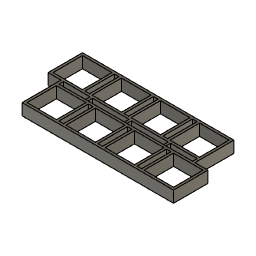
Macropad_V1_Plate (Autodesk Fusion 360 design; units mm, degrees)
Autodesk Fusion 360 part; units mm, degrees
sketch "Sketch1" plane through (0, 0, 0) normal (0, 0, 1) x (1, 0, 0)
  line L0 (0, 0) -> (80.3, 0)
  line L1 (80.3, 0) -> (80.3, 35.85)
  line L2 (80.3, 35.85) -> (0, 35.85)
  line L3 (0, 35.85) -> (0, 0)
  line L4 (1.2, 34.65) -> (15.6, 34.65)
  line L5 (15.6, 34.65) -> (15.6, 20.25)
  line L6 (15.6, 20.25) -> (1.2, 20.25)
  line L7 (1.2, 20.25) -> (1.2, 34.65)
  line L8 (20.25, 20.25) -> (20.25, 34.65)
  line L9 (20.25, 34.65) -> (34.65, 34.65)
  line L10 (34.65, 34.65) -> (34.65, 20.25)
  line L11 (34.65, 20.25) -> (20.25, 20.25)
  line L12 (39.3, 20.25) -> (39.3, 34.65)
  line L13 (39.3, 34.65) -> (53.7, 34.65)
  line L14 (53.7, 34.65) -> (53.7, 20.25)
  line L15 (53.7, 20.25) -> (39.3, 20.25)
  line L16 (58.35, 20.25) -> (58.35, 34.65)
  line L17 (58.35, 34.65) -> (72.75, 34.65)
  line L18 (72.75, 34.65) -> (72.75, 20.25)
  line L19 (72.75, 20.25) -> (58.35, 20.25)
  line L20 (7.55, 1.2) -> (7.55, 15.6)
  line L21 (7.55, 15.6) -> (21.95, 15.6)
  line L22 (21.95, 15.6) -> (21.95, 1.2)
  line L23 (21.95, 1.2) -> (7.55, 1.2)
  line L24 (26.6, 1.2) -> (26.6, 15.6)
  line L25 (26.6, 15.6) -> (41, 15.6)
  line L26 (41, 15.6) -> (41, 1.2)
  line L27 (41, 1.2) -> (26.6, 1.2)
  line L28 (45.65, 1.2) -> (45.65, 15.6)
  line L29 (45.65, 15.6) -> (60.05, 15.6)
  line L30 (60.05, 15.6) -> (60.05, 1.2)
  line L31 (60.05, 1.2) -> (45.65, 1.2)
  line L32 (64.7, 1.2) -> (64.7, 15.6)
  line L33 (64.7, 15.6) -> (79.1, 15.6)
  line L34 (79.1, 15.6) -> (79.1, 1.2)
  line L35 (79.1, 1.2) -> (64.7, 1.2)
  line L36 (19.05, 34.65) -> (16.8, 34.65)
  line L37 (16.8, 34.65) -> (16.8, 20.25)
  line L38 (16.8, 20.25) -> (19.05, 20.25)
  line L39 (19.05, 20.25) -> (19.05, 34.65)
  line L40 (35.85, 34.65) -> (35.85, 20.25)
  line L41 (35.85, 20.25) -> (38.1, 20.25)
  line L42 (38.1, 20.25) -> (38.1, 34.65)
  line L43 (38.1, 34.65) -> (35.85, 34.65)
  line L44 (54.9, 34.65) -> (54.9, 20.25)
  line L45 (54.9, 20.25) -> (57.15, 20.25)
  line L46 (57.15, 20.25) -> (57.15, 34.65)
  line L47 (57.15, 34.65) -> (54.9, 34.65)
  line L48 (25.4, 15.6) -> (23.15, 15.6)
  line L49 (23.15, 15.6) -> (23.15, 1.2)
  line L50 (23.15, 1.2) -> (25.4, 1.2)
  line L51 (25.4, 1.2) -> (25.4, 15.6)
  line L52 (42.2, 15.6) -> (42.2, 1.2)
  line L53 (42.2, 1.2) -> (44.45, 1.2)
  line L54 (44.45, 1.2) -> (44.45, 15.6)
  line L55 (44.45, 15.6) -> (42.2, 15.6)
  line L56 (61.25, 15.6) -> (61.25, 1.2)
  line L57 (61.25, 1.2) -> (63.5, 1.2)
  line L58 (63.5, 1.2) -> (63.5, 15.6)
  line L59 (63.5, 15.6) -> (61.25, 15.6)
  line L60 (72.75, 19.05) -> (7.55, 19.05)
  line L61 (7.55, 19.05) -> (7.55, 16.8)
  line L62 (7.55, 16.8) -> (72.75, 16.8)
  line L63 (72.75, 16.8) -> (72.75, 19.05)
  line L64 (80.3, 35.85) -> (73.95, 35.85)
  line L65 (73.95, 35.85) -> (73.95, 16.8)
  line L66 (73.95, 16.8) -> (80.3, 16.8)
  line L67 (80.3, 16.8) -> (80.3, 35.85)
  line L68 (0, 0) -> (6.35, 0)
  line L69 (6.35, 0) -> (6.35, 19.05)
  line L70 (6.35, 19.05) -> (0, 19.05)
  line L71 (0, 19.05) -> (0, 0)
  line L72 (21.7, 19.05) -> (20.5, 19.05)
  line L73 (20.5, 19.05) -> (20.5, 16.8018)
  line L74 (20.5, 16.8018) -> (21.7, 16.8018)
  line L75 (21.7, 16.8018) -> (21.7, 19.05)
  line L76 (40.75, 16.8018) -> (40.75, 19.05)
  line L77 (40.75, 19.05) -> (39.55, 19.05)
  line L78 (39.55, 19.05) -> (39.55, 16.8018)
  line L79 (39.55, 16.8018) -> (40.75, 16.8018)
  line L80 (59.8, 16.8018) -> (59.8, 19.05)
  line L81 (59.8, 19.05) -> (58.6, 19.05)
  line L82 (58.6, 19.05) -> (58.6, 16.8018)
  line L83 (58.6, 16.8018) -> (59.8, 16.8018)
  dimension "d6" = 14.4
  dimension "d7" = 14.4
  dimension "d12" = 19.05
  dimension "d13" = 0
  dimension "d14" = 14.4
  dimension "d15" = 14.4
  dimension "d16" = 19.05
  dimension "d17" = 6.35
  dimension "d20" = 19.05
  dimension "d21" = 0
  dimension "d22" = 1.2
  dimension "d23" = 1.2
  dimension "d24" = 1.2
  dimension "d25" = 1.2
  dimension "d37" = 1.2
  dimension "d39" = 1.2
  dimension "d42" = 19.05
  dimension "d43" = 0
  dimension "d45" = 1.2
  dimension "d46" = 1.2
  dimension "d49" = 19.05
  dimension "d50" = 0
  dimension "d54" = 1.2
  dimension "d55" = 1.2
  dimension "d57" = 1.2
  dimension "d59" = 1.2
  dimension "d60" = 1.2
  dimension "d61" = 0.25
  dimension "d64" = 19.05
  dimension "d65" = 0
  constraint horizontal L0
  constraint vertical L1
  constraint horizontal L2
  constraint vertical L3
  constraint coincident L0.start L3.end
  constraint horizontal L4
  constraint vertical L5
  constraint horizontal L6
  constraint vertical L7
  constraint horizontal L21
  constraint vertical L22
  constraint horizontal L23
  constraint vertical L20
  constraint horizontal L36
  constraint vertical L37
  constraint horizontal L38
  constraint vertical L39
  constraint collinear L4 L36
  constraint collinear L6 L38
  constraint horizontal L48
  constraint vertical L49
  constraint horizontal L50
  constraint vertical L51
  constraint collinear L21 L48
  constraint collinear L23 L50
  constraint horizontal L60
  constraint vertical L61
  constraint horizontal L62
  constraint vertical L63
  constraint collinear L18 L63
  constraint collinear L20 L61
  constraint horizontal L64
  constraint vertical L65
  constraint horizontal L66
  constraint vertical L67
  constraint collinear L62 L66
  constraint horizontal L68
  constraint vertical L69
  constraint horizontal L70
  constraint vertical L71
  constraint collinear L60 L70
  constraint horizontal L72
  constraint vertical L73
  constraint horizontal L74
  constraint vertical L75
  constraint coincident L60 L72.start
  measures "d6" distance of L4.start L4.end
  measures "d7" distance of L4.start L6.end
  measures "d14" distance of L20.end L21.end
  measures "d15" distance of L20.start L20.end
  measures "d16" vertical distance of L6.end L20.start
  measures "d17" horizontal distance of L6.end L20.start
  measures "d22" horizontal distance of L2.end L4.start
  measures "d23" vertical distance of L2.end L4.start
  measures "d24" vertical distance of L0.start L20.start
  measures "d25" horizontal distance of L0.end L34.end
  measures "d37" horizontal distance of L4.end L36.end
  measures "d39" distance of L8.end L36.start
  measures "d45" distance of L21.end L48.end
  measures "d46" distance of L24.end L48.start
  measures "d54" distance of L18.end L60.start
  measures "d55" vertical distance of L33.end L62.end
  measures "d57" distance of L18 L65
  measures "d59" distance of L20 L69
  measures "d60" distance of L72.start L72.end
  measures "d61" distance of L8 L73
extrude "Extrude3" add sketch "Sketch1" along normal blind 5.6 contours L0 L1 L2 L3 L65 L66 L69 L70 | L60 L80 L81 L82 L83 | L60 L76 L77 L78 L79 | L60 L72 L73 L74 L75
named bodies: "Plate"
